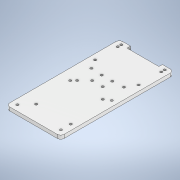
# Autodesk Inventor part: Top plate
Saved by Autodesk Inventor 2022.6 (Build 266554000, 554)
## iProperties
Created: 2024-10-12
Part Number: Top plate
Material: PBT Plastic
Document SubType Name: Modeling
Designer: Zhong
Density: 1.31 g/cm^3
Appearance: Smooth - White
Author: Zhong
Autodesk Inventor part; units mm, degrees
ref_plane "YZ Plane" through (0, 0, 0) normal (1, 0, 0) x (0, 1, 0)
ref_plane "XZ Plane" through (0, 0, 0) normal (0, 1, 0) x (-1, 0, 0)
ref_plane "XY Plane" through (0, 0, 0) normal (0, 0, 1) x (1, 0, 0)
sketch "Sketch1" plane through (0, 0, 0) normal (0, 1, 0) x (-1, 0, 0)
  line L0 (38.5, 80) -> (-38.5, 80)
  line L1 (-38.5, 80) -> (-38.5, -80)
  line L2 (-38.5, -80) -> (38.5, -80)
  line L3 (38.5, -80) -> (38.5, 80)
  line L4 (38.5, 0) -> (-38.5, 0) construction
  line L5 (0, 80) -> (0, -80) construction
  line L6 (-22.5, -80) -> (22.5, -80)
  line L7 (22.5, -80) -> (22.5, -75)
  line L8 (22.5, -75) -> (-22.5, -75)
  line L9 (-22.5, -75) -> (-22.5, -80)
  point P0 (0, 0)
  point P1 (0, 0)
  dimension "d0" = 77
  dimension "d1" = 160
  dimension "d64" = 45
  dimension "d65" = 5
  constraints: 20 end point, 5 midpoint, 4 parallel, 2 horizontal, 2 perpendicular, 1 coincident, 1 point on line, 1 other
  measures "d0" distance of L0.start L0.end
  measures "d1" distance of L2.end L0.start
  measures "d64" distance of L7.end L8.end
  measures "d65" distance of L6.end L7.end
extrude "Extrusion1" add sketch "Sketch1" along normal blind 5 contours L3 L2 L7 L8 L9 L1 L0
fillet "Fillet1" radius 5 4 edges at (-38.5, 2.5, 80) (38.5, 2.5, 80) (38.5, 2.5, -80) (-38.5, 2.5, -80)
sketch "Sketch3" plane through (0, 5, 0) normal (0, 1, 0) x (1, 0, 0)
  line L0 (33.5, 80) -> (-33.5, 80) construction
  line L1 (-30.75, -72) -> (-30.75, 75) construction
  line L2 (-30.75, 75) -> (30.75, 75) construction
  line L3 (30.75, 75) -> (30.75, -72) construction
  line L4 (30.75, -72) -> (-30.75, -72) construction
  line L5 (0, 112) -> (0, -112) construction
  line L6 (-33.5, -80) -> (33.5, -80) projected
  line L7 (38.5, -75) -> (38.5, 75) projected
  line L8 (-38.5, 75) -> (-38.5, -75) projected
  point P0 (0, 0)
  point P1 (0, -72)
  point P2 (0, -80)
  dimension "d15" = 147
  dimension "d18" = 8
  dimension "d56" = 61.5
  constraints: 8 end point, 2 midpoint, 2 parallel, 1 perpendicular, 1 point on line, 1 vertical alignment
  measures "d15" distance of L1.end L1.start
  measures "d18" distance of point (0, -80) point (0, -72)
  measures "d56" distance between parallel lines of L3 L1
hole "Brass stands" at (-30.75, 5, 72) at (30.75, 5, 72) at (30.75, 5, -75) at (-30.75, 5, -75) direction (0, -1, 0) diameter 3.4 end through all
sketch "Sketch5" plane through (0, 5, 0) normal (0, 1, 0) x (1, 0, 0)
  line L0 (-23, -5) -> (23, -5) construction
  line L1 (23, -5) -> (23, 25) construction
  line L2 (23, 25) -> (-23, 25) construction
  line L3 (-23, 25) -> (-23, -5) construction
  line L4 (-23, -5) -> (23, 25) construction
  line L5 (23, -5) -> (-23, 25) construction
  line L6 (0, 112) -> (0, -112) construction
  line L7 (33.5, 80) -> (-33.5, 80) construction
  point P0 (0, 0)
  point P1 (0, 10)
  point P2 (0, 10)
  point P3 (-23, 25)
  point P4 (23, 25)
  dimension "d31" = 30
  dimension "d32" = 46
  dimension "d33" = 55
  constraints: 12 end point, 4 coincident, 3 midpoint, 2 parallel, 1 horizontal, 1 perpendicular, 1 point on line
  measures "d31" distance of L2.end L0.start
  measures "d32" distance of L0.start L0.end
  measures "d33" distance between parallel lines of L7 L2
hole "Battery mount" at (-23, 5, 5) at (-23, 5, -25) at (23, 5, -25) at (23, 5, 5) direction (0, -1, 0) diameter 3.4 end through all
sketch "Sketch7" plane through (0, 5, 0) normal (0, 1, 0) x (1, 0, 0)
  line L0 (7.5, 24) -> (-7.5, 24) construction
  line L1 (-7.5, 24) -> (-7.5, 10.5) construction
  line L2 (-7.5, 10.5) -> (7.5, 10.5) construction
  line L3 (7.5, 10.5) -> (7.5, 24) construction
  line L4 (7.5, 24) -> (-7.5, 10.5) construction
  line L5 (-7.5, 24) -> (7.5, 10.5) construction
  line L6 (33.5, 80) -> (22.5, 80) construction
  line L7 (38.5, -75) -> (38.5, 75) construction
  line L8 (22.5, 75) -> (-22.5, 75) construction
  line L9 (0, 112) -> (0, -112) construction
  point P0 (0, 0)
  point P1 (0, 17.25)
  point P2 (54.473, 10.5)
  point P3 (0, 24)
  point P4 (0, 17.25)
  dimension "d66" = 13.5
  dimension "d67" = 15
  dimension "d71" = 51
  constraints: 12 end point, 4 midpoint, 3 coincident, 2 parallel, 1 horizontal, 1 perpendicular, 1 point on line, 2 other
  measures "d66" distance of L2.end L0.start
  measures "d67" distance of L1.end L2.end
  measures "d71" distance between parallel lines of L8 L0
hole "pi cam" at (7.5, 5, -24) at (7.5, 5, -10.5) at (54.473, 5, -10.5) at (-7.5, 5, -24) at (-7.5, 5, -10.5) direction (0, -1, 0) diameter 3.4 end through all
sketch "Sketch8" plane through (0, 5, 0) normal (0, 1, 0) x (1, 0, 0)
  circle A0 centre (-7.5, 24) radius 1.7 projected
  circle A1 centre (7.5, 10.5) radius 1.7 projected
  circle A2 centre (7.5, 24) radius 1.7 projected
  circle A3 centre (-7.5, 10.5) radius 1.7 projected
  circle A4 centre (23, 25) radius 1.7 projected
  circle A5 centre (-23, -5) radius 1.7 projected
  circle A6 centre (-23, 25) radius 1.7 projected
  circle A7 centre (23, -5) radius 1.7 projected
  circle A8 centre (30.75, 75) radius 1.7 projected
  circle A9 centre (-30.75, -72) radius 1.7 projected
  circle A10 centre (30.75, -72) radius 1.7 projected
  circle A11 centre (-30.75, 75) radius 1.7 projected
  arc A12 (-33.5, 80) -> (-38.5, 75) centre (-33.5, 75) ccw projected
  line L0 (-38.5, 75) -> (-38.5, -75) projected
  arc A13 (-38.5, -75) -> (-33.5, -80) centre (-33.5, -75) ccw projected
  line L1 (-33.5, -80) -> (33.5, -80) projected
  arc A14 (33.5, -80) -> (38.5, -75) centre (33.5, -75) ccw projected
  line L2 (38.5, -75) -> (38.5, 75) projected
  arc A15 (38.5, 75) -> (33.5, 80) centre (33.5, 75) ccw projected
  line L3 (33.5, 80) -> (22.5, 80) projected
  line L4 (22.5, 80) -> (22.5, 75) projected
  line L5 (22.5, 75) -> (-22.5, 75) projected
  line L6 (-22.5, 75) -> (-22.5, 80) projected
  line L7 (-22.5, 80) -> (-33.5, 80) projected
  line L8 (30.75, 0) -> (-18.25, 0) construction
  line L9 (-18.25, 0) -> (-18.25, -58) construction
  line L10 (-18.25, -58) -> (30.75, -58) construction
  line L11 (30.75, -58) -> (30.75, 0) construction
  line L12 (30.75, 0) -> (-18.25, -58) construction
  line L13 (-18.25, 0) -> (30.75, -58) construction
  point P0 (0, 0)
  point P1 (6.25, -29)
  dimension "d79" = 49
  dimension "d80" = 58
  dimension "d81" = 22
  dimension "d82" = 7.75
  constraints: 12 end point, 4 coincident, 2 midpoint, 2 parallel, 1 horizontal, 1 perpendicular
  measures "d79" distance of L8.start L8.end
  measures "d80" distance of L8.end L9.end
  measures "d81" distance between parallel lines of L1 L10
  measures "d82" distance between parallel lines of L2 L11
hole "raspberry pi" at (30.75, 5, 0) at (30.75, 5, 58) at (-18.25, 5, 58) at (-18.25, 5, 0) direction (0, -1, 0) diameter 3.4 end through all
sketch "buck convertor" plane through (0, 5, 0) normal (0, 1, 0) x (1, 0, 0)
  line L0 (38.5, -75) -> (38.5, 75) projected
  circle A0 centre (-18.25, -58) radius 1.7 projected
  circle A1 centre (30.75, 0) radius 1.7 projected
  circle A2 centre (30.75, -58) radius 1.7 projected
  circle A3 centre (-18.25, 0) radius 1.7 projected
  circle A4 centre (-7.5, 24) radius 1.7 projected
  circle A5 centre (7.5, 10.5) radius 1.7 projected
  circle A6 centre (7.5, 24) radius 1.7 projected
  circle A7 centre (-7.5, 10.5) radius 1.7 projected
  circle A8 centre (23, 25) radius 1.7 projected
  circle A9 centre (-23, -5) radius 1.7 projected
  circle A10 centre (-23, 25) radius 1.7 projected
  circle A11 centre (23, -5) radius 1.7 projected
  circle A12 centre (30.75, 75) radius 1.7 projected
  circle A13 centre (-30.75, -72) radius 1.7 projected
  circle A14 centre (30.75, -72) radius 1.7 projected
  circle A15 centre (-30.75, 75) radius 1.7 projected
  arc A16 (-33.5, 80) -> (-38.5, 75) centre (-33.5, 75) ccw projected
  line L1 (-38.5, 75) -> (-38.5, -75) projected
  arc A17 (-38.5, -75) -> (-33.5, -80) centre (-33.5, -75) ccw projected
  line L2 (-33.5, -80) -> (33.5, -80) projected
  arc A18 (33.5, -80) -> (38.5, -75) centre (33.5, -75) ccw projected
  line L3 (38.5, -75) -> (38.5, 75) projected
  arc A19 (38.5, 75) -> (33.5, 80) centre (33.5, 75) ccw projected
  line L4 (33.5, 80) -> (22.5, 80) projected
  line L5 (22.5, 80) -> (22.5, 75) projected
  line L6 (22.5, 75) -> (-22.5, 75) projected
  line L7 (-22.5, 75) -> (-22.5, 80) projected
  line L8 (-22.5, 80) -> (-33.5, 80) projected
  line L9 (30.75, 70) -> (-30.75, 70) construction
  line L10 (-30.75, 70) -> (-30.75, 38) construction
  line L11 (-30.75, 38) -> (30.75, 38) construction
  line L12 (30.75, 38) -> (30.75, 70) construction
  line L13 (30.75, 70) -> (-30.75, 38) construction
  line L14 (-30.75, 70) -> (30.75, 38) construction
  line L15 (0, 113.4497) -> (0, -113.4497) projected
  point P0 (0, 0)
  point P1 (0, 54)
  point P2 (0, 54)
  dimension "d90" = 32
  dimension "d98" = 10
  constraints: 12 end point, 4 coincident, 3 midpoint, 2 parallel, 1 horizontal, 1 perpendicular, 1 point on line, 1 vertical alignment
  measures "d90" distance of L11.end L9.start
  measures "d98" distance between parallel lines of L4 L9
hole "Hole7" at (30.75, 5, -38) at (-30.75, 5, -38) at (30.75, 5, -70) at (-30.75, 5, -70) direction (0, -1, 0) diameter 3.4 end through all
body "Solid1"
